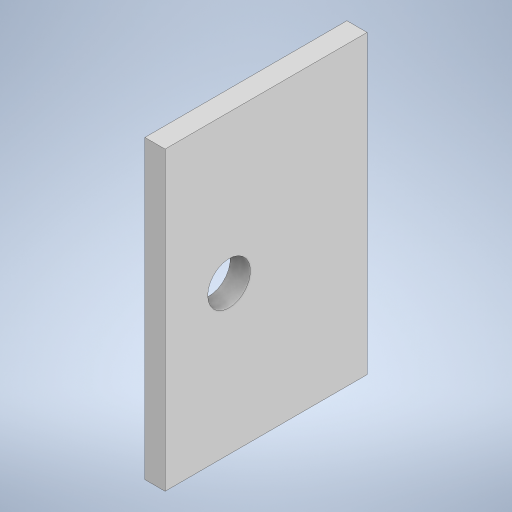
# Autodesk Inventor part: motor_base
Saved by Autodesk Inventor 2023 (Build 270158000, 158)
## iProperties
Created: 2023-04-09
Part Number: motor_base
Material: Generic
Document SubType Name: Modeling
Designer: Nikhil
Density: 1 g/cm^3
Appearance: Default
Author: Nikhil
Autodesk Inventor part; units mm, degrees
ref_plane "YZ Plane" through (0, 0, 0) normal (1, 0, 0) x (0, 1, 0)
ref_plane "XZ Plane" through (0, 0, 0) normal (0, 1, 0) x (-1, 0, 0)
ref_plane "XY Plane" through (0, 0, 0) normal (0, 0, 1) x (1, 0, 0)
sketch "Sketch1" plane through (0, 0, 0) normal (1, 0, 0) x (0, 1, 0)
  line L0 (0, 0) -> (88, 0)
  line L1 (88, 0) -> (88, 60)
  line L2 (88, 60) -> (0, 60)
  line L3 (0, 60) -> (0, 0)
  dimension "d0" = 88
  dimension "d1" = 60
  constraints: 8 end point, 2 parallel, 1 horizontal, 1 perpendicular
  measures "d0" distance of L2.end L1.end
  measures "d1" distance of L1.end L0.end
extrude "Extrusion1" add sketch "Sketch1" along normal blind 6
sketch "Sketch2" plane through (0, 0, 0) normal (-1, 0, 0) x (0, 0, 1)
  line L0 (60, 0) -> (0, 0) projected
  line L1 (0, 0) -> (0, 88) projected
  circle A0 centre (41, 44) radius 6.35
  dimension "d4" = 44
  dimension "d5" = 41
  dimension "d6" = 12.7
  constraints: 1 centre point, 1 coincident
  measures "d4" distance from line of L0 point (41, 44)
  measures "d5" distance from line of L1 point (41, 44)
  measures "d6" diameter of A0
extrude "Extrusion2" cut sketch "Sketch2" against normal blind 6
body "Solid1"
